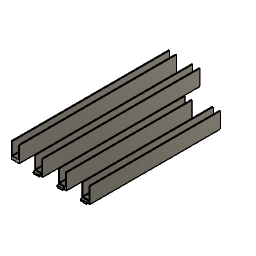
Correção Janela traseiro saveiro v3 (Autodesk Fusion 360 design; units mm, degrees)
Autodesk Fusion 360 part; units mm, degrees
sketch "Esboço1" plane through (0, 0, 0) normal (0, 1, 0) x (1, 0, 0)
  line L0 (0, 0) -> (5, 0)
  line L1 (5, 0) -> (5, -10)
  line L2 (5, -10) -> (0, -10)
  line L3 (0, -10) -> (0, 0)
  dimension "d1" = 10
  dimension "d2" = 5
  constraint horizontal L0
  constraint vertical L1
  constraint horizontal L2
  constraint vertical L3
  constraint coincident L0.start L3.end
  measures "d1" distance of L0.start L2.end
  measures "d2" distance of L0.start L0.end
extrude "Extrusão1" add sketch "Esboço1" along normal blind 363 makes body 1
ref_plane "Plano de trabalho1" through (2.5, 0, 0) normal (1, 0, 0) x (0, 1, 0)
sketch "Esboço2" plane through (2.5, 0, 0) normal (1, 0, 0) x (0, 1, 0)
  line L0 (0, 10) -> (364, 10)
  line L1 (364, 10) -> (364, 2)
  line L2 (364, 2) -> (0, 2)
  line L3 (0, 2) -> (0, 10)
  dimension "d6" = 364
  dimension "d7" = 8
  dimension "d8" = 2
  constraint horizontal L0
  constraint vertical L1
  constraint horizontal L2
  constraint vertical L3
  measures "d6" distance of L0.start L0.end
  measures "d7" distance of L0.start L2.end
  measures "d8" distance of origin L2.end
extrude "Extrusão2" cut sketch "Esboço2" along normal mid plane 4.02 bodies 1
fillet "Arredondamento1" radius 0.2 1 edges at (4.755, 0, 10) on bodies 1
fillet "Arredondamento2" radius 0.2 1 edges at (0.245, 0, 10) on bodies 1
fillet "Arredondamento3" radius 0.2 1 edges at (4.755, 363, 10) on bodies 1
fillet "Arredondamento4" radius 0.2 1 edges at (0.245, 363, 10) on bodies 1
fillet "Arredondamento5" radius 0.2 1 edges at (4.51, 181.5, 2) on bodies 1
fillet "Arredondamento6" radius 0.2 1 edges at (0.49, 181.5, 2) on bodies 1
ref_plane "Plano de trabalho8" through (0, 100, 0) normal (0, 1, 0) x (0, 0, 1)
sketch "Esboço13" plane through (5, 0, 0) normal (1, 0, 0) x (0, 1, 0)
  arc A0 (363, 9.8) -> (362.8, 10) centre (362.8, 9.8) ccw
  line L0 (362.8, 10) -> (0.2, 10)
  arc A1 (0.2, 10) -> (0, 9.8) centre (0.2, 9.8) ccw
  line L1 (0, 9.8) -> (0, 0)
  line L2 (0, 0) -> (363, 0)
  line L3 (363, 0) -> (363, 9.8)
  line L4 (100, 13) -> (100, -3)
  dimension "d37" = 100
  constraint vertical L4
  measures "d37" distance of L1 L4
split "Dividir3" by curves path "Esboço13" along L4 bodies 1 makes body 2 at (5, 33.4, 3.3333)
move_body "Mover1" bodies 2 to x (1, 0, 0) y (0, 1, 0) z (0, 0, 1) at (0, -5, 0)
box "Primitiva de caixa1" add length 0.9159 width 3.9818 height 1.5 placed x (0, 0, -1) y (1, 0, 0) z (0, -1, 0) at (0.3, 100, 1.5) bodies 1
move_body "Mover2" bodies 2 to x (1, 0, 0) y (0, 1, 0) z (0, 0, 1) at (0, 5, 0)
combine "Combinar1" operation cut target body 2 tool bodies 1 keep tools
sketch "Esboço15" plane through (5, 0, 0) normal (1, 0, 0) x (0, 1, 0)
  line L0 (100, 10) -> (100, 0)
  line L1 (100, 0) -> (363, 0)
  line L2 (363, 0) -> (363, 9.8)
  arc A0 (363, 9.8) -> (362.8, 10) centre (362.8, 9.8) ccw
  line L3 (362.8, 10) -> (100, 10)
  line L4 (200, 15) -> (200, -5)
  dimension "d43" = 100
  constraint vertical L4
  measures "d43" distance of L0 L4
split "Dividir4" by curves path "Esboço15" along L4 bodies 1 makes body 3 at (5, 133.3333, 3.3333)
box "Primitiva de caixa2" add length 1 width 3.5 height 1.5 placed x (0, 0, -1) y (1, 0, 0) z (0, -1, 0) at (0.5, 200, 1.5) bodies 1
combine "Combinar2" operation cut target body 3 tool bodies 1 keep tools
sketch "Esboço17" plane through (5, 0, 0) normal (1, 0, 0) x (0, 1, 0)
  line L0 (200, 10) -> (200, 0)
  line L1 (200, 0) -> (363, 0)
  line L2 (363, 0) -> (363, 9.8)
  arc A0 (363, 9.8) -> (362.8, 10) centre (362.8, 9.8) ccw
  line L3 (362.8, 10) -> (200, 10)
  line L4 (280, 21) -> (280, -7)
  dimension "d49" = 80
  constraint vertical L4
  measures "d49" distance of L0 L4
split "Dividir5" by curves path "Esboço17" along L4 bodies 1 makes body 4 at (5, 253.3333, 3.3333)
box "Primitiva de caixa3" add length 1 width 3.8 height 1.5 placed x (0, 0, -1) y (1, 0, 0) z (0, -1, 0) at (0.5, 280, 1.5) bodies 1
combine "Combinar3" operation cut target body 4 tool bodies 1 keep tools
move_body "Mover4" bodies 2 to x (1, 0, 0) y (0, 1, 0) z (0, 0, 1) at (-35, 0, 0)
move_body "Mover5" bodies 3 to x (1, 0, 0) y (0, 1, 0) z (0, 0, 1) at (-20, -100, 0)
move_body "Mover6" bodies 4 to x (1, 0, 0) y (0, 1, 0) z (0, 0, 1) at (-5, -200, 0)
move_body "Mover7" bodies 1 to x (1, 0, 0) y (0, 1, 0) z (0, 0, 1) at (10, -280, 0)
